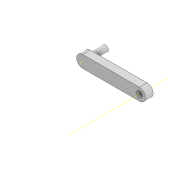
# Autodesk Inventor part: Manivela
Saved by Autodesk Inventor 2021 (Build 250183000, 183)
## iProperties
Created: 2021-07-04
Part Number: Manivela
Material: Generic
Document SubType Name: Modeling
Designer: Santiago
Density: 1 g/cm^3
Appearance: Default
Mass: 14.5133 g
Surface Area: 54.5823 cm^2
Volume: 14.5133 cm^3
Author: Santiago
Autodesk Inventor part; units mm, degrees
ref_plane "XZ Plane" through (0, 0, 0) normal (0, 1, 0) x (-1, 0, 0)
ref_plane "XY Plane" through (0, 0, 0) normal (0, 0, 1) x (1, 0, 0)
sketch "Sketch1" plane through (0, 0, 0) normal (0, 0, 1) x (1, 0, 0)
  circle A0 centre (0, 0) radius 8
  dimension "d0" = 16
  constraints: 1 centre point, 1 coincident
  measures "d0" diameter of A0
extrude "Extrusion1" add sketch "Sketch1" along normal blind 10
ref_plane "Work Plane1" through (8, 0, 0) normal (1, 0, 0) x (0, 1, 0)
sketch "Sketch2" plane through (8, 0, 0) normal (1, 0, 0) x (0, 1, 0)
  line L0 (8, 10) -> (-8, 10) projected
  line L1 (8, 0) -> (-8, 0) projected
  line L2 (8, 0) -> (-8, 0) projected
  line L3 (-8, 10) -> (8, 10)
  line L4 (8, 10) -> (8, 0)
  line L5 (8, 0) -> (-8, 0)
  line L6 (-8, 0) -> (-8, 10)
  line L7 (-8, 10) -> (8, 0) construction
  line L8 (8, 10) -> (-8, 0) construction
  point P0 (0, 0)
  point P1 (0, 5)
  constraints: 12 end point, 2 midpoint, 2 parallel, 1 horizontal, 1 perpendicular
extrude "Extrusion2" add sketch "Sketch2" along normal blind 67 and the other way blind 8
sketch "Sketch3" plane through (0, 0, 0) normal (0, 0, -1) x (-1, 0, 0)
  line L0 (0, 0) -> (-75, 0)
  line L1 (-75, -8) -> (-75, 8) projected
  circle A0 centre (-75, 0) radius 8
  dimension "d8" = 75
  constraints: 2 end point, 1 coincident, 1 midpoint, 3 other
  measures "d8" distance of L0.start L0.end
extrude "Extrusion3" add sketch "Sketch3" against normal blind 10 contours L1 A0
sketch "Sketch4" plane through (0, 0, 0) normal (0, 0, -1) x (-1, 0, 0)
  line L0 (0, 0) -> (-75, 0)
  line L1 (0, -8) -> (-75, -8) projected
  line L2 (0, 0) -> (75, 0) construction
  circle A0 centre (-75, 0) radius 4
  circle A1 centre (0, 0) radius 4
  dimension "d11" = 75
  dimension "d12" = 180
  dimension "d14" = 8
  dimension "d15" = 8
  constraints: 4 end point, 2 centre point, 2 coincident, 1 collinear, 1 horizontal, 1 parallel, 1 point on line
  measures "d11" distance of L0.start L0.end
  measures "d12" angle of L0 L2
  measures "d14" diameter of A0
  measures "d15" diameter of A1
extrude "Extrusion4" add sketch "Sketch4" along normal blind 20 contours A1
hole "Hole1" at (75, 0, 0) direction (0, 0, 1) diameter 8 end through all
ref_plane "Work Plane2" through (68, 0, 0) normal (1, 0, 0) x (0, 1, 0)
sketch "Sketch6" plane through (68, 0, 0) normal (1, 0, 0) x (0, 1, 0)
  line L0 (-8, 0) -> (-8, 10) projected
  line L1 (8, 7.5) -> (-8, 7.5)
  line L2 (-8, 7.5) -> (-8, 2.5)
  line L3 (-8, 2.5) -> (8, 2.5)
  line L4 (8, 2.5) -> (8, 7.5)
  line L5 (8, 7.5) -> (-8, 2.5) construction
  line L6 (-8, 7.5) -> (8, 2.5) construction
  point P0 (0, 0)
  point P1 (0, 5)
  dimension "d28" = 5
  constraints: 12 end point, 2 midpoint, 2 parallel, 1 horizontal, 1 perpendicular, 1 point on line
  measures "d28" distance of L2.end L1.end
extrude "Extrusion6" [suppressed]
body "Solid1"
